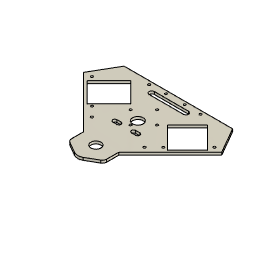
侧板1-正面 v9 (Autodesk Fusion 360 design; units mm, degrees)
Autodesk Fusion 360 part; units mm, degrees
sketch "草图1" plane through (0, 0, 0) normal (0, 0, 1) x (1, 0, 0)
  line L0 (-54.1241, 76.0619) -> (-2.5053, 24.4431)
  line L1 (93.1135, 76.0619) -> (41.4947, 24.4431)
  line L2 (16.6481, 16.6481) -> (19.4947, 16.6481)
  line L3 (-43.8746, 113.133) -> (82.8641, 113.133)
  line L4 (19.4947, 16.6481) -> (19.4947, 38.6817) construction
  line L5 (-2.5053, 4.4431) -> (23.0093, 4.4431) construction
  line L6 (-54.1241, 76.0619) -> (-61.1951, 83.133)
  line L7 (-61.1951, 83.133) -> (-43.8746, 113.133)
  line L8 (-61.1951, 83.133) -> (-22.8991, 83.133) construction
  line L9 (100.1846, 83.133) -> (82.8641, 113.133)
  line L10 (93.1135, 76.0619) -> (100.1846, 83.133)
  line L11 (-2.5053, 24.4431) -> (-1.091, 23.0289)
  line L12 (-1.091, 23.0289) -> (-1.091, 6.0289)
  line L13 (-1.091, 6.0289) -> (19.4947, -5.8563)
  line L14 (19.4947, -5.8563) -> (19.4947, 1) construction
  line L15 (40.0805, 6.0289) -> (19.4947, -5.8563)
  line L16 (40.0805, 23.0289) -> (40.0805, 6.0289)
  line L17 (41.4947, 24.4431) -> (40.0805, 23.0289)
  dimension "d8" = 20
  dimension "d9" = 73
  dimension "d75" = 10
  dimension "d76" = 60
  dimension "d81" = 2
  dimension "d82" = 17
  dimension "d96" = 30
  constraint perpendicular L0 L1
  constraint horizontal L2
  constraint perpendicular L2 L4
  constraint symmetric L0.end L4 L1.end
  constraint horizontal L5
  constraint equal L0 L1
  constraint parallel L0 L6
  constraint horizontal L8
  constraint symmetric L0.start L4 L1.start
  constraint symmetric L4 L6.end L9.start
  constraint symmetric L4 L3.start L3.end
  constraint parallel L0 L11
  constraint perpendicular L5 L12
  constraint vertical L14
  constraint symmetric L0.end L14 L1.end
  constraint symmetric L11.end L14 L16.start
  constraint symmetric L12.end L14 L15.start
  constraint symmetric L13.end L14 L15.end
  measures "d8" distance of L0.end L5.start
  measures "d9" distance of L0.start L0.end
  measures "d75" distance of L0.start L6.end
  measures "d76" angle of L7 L8
  measures "d81" distance of L0.end L11.end
  measures "d82" distance of L11.end L12.end
  measures "d96" distance of L3 L8
extrude "拉伸1" add sketch "草图1" along normal blind 3
sketch "草图2" plane through (0, 0, 3) normal (0, 0, 1) x (-1, 0, 0)
  line L0 (61.1951, -83.133) -> (1.091, -23.0289)
  line L1 (-40.0805, -23.0289) -> (-100.1846, -83.133)
  line L2 (-82.8641, -113.133) -> (43.8746, -113.133)
  line L3 (61.1951, -83.133) -> (56.2454, -88.0827) construction
  line L4 (56.2454, -88.0827) -> (52.0027, -83.8401) construction
  circle A0 centre (52.0027, -83.8401) radius 1.3
  line L5 (52.0027, -83.8401) -> (22.1494, -53.9867) construction
  circle A1 centre (22.1494, -53.9867) radius 1.3
  line L6 (-19.4947, 8.2586) -> (-19.4947, -40) construction
  circle A2 centre (-61.1389, -53.9867) radius 1.3
  circle A3 centre (-90.9922, -83.8401) radius 1.3
  line L7 (-19.4947, -113.133) -> (-19.4947, -109.133) construction
  line L8 (-19.4947, -109.133) -> (-19.4947, -87.1743)
  line L9 (-19.4947, -87.1743) -> (-19.4947, -80.1743) construction
  circle A4 centre (-19.4947, -16.9209) radius 5.95
  line L10 (-90.9922, -83.8401) -> (-75.2591, -68.107) construction
  line L11 (-75.2591, -68.107) -> (-78.0875, -65.2785) construction
  line L12 (-78.0875, -65.2785) -> (-89.7548, -76.9458)
  line L13 (-89.7548, -76.9458) -> (-64.2989, -102.4016)
  line L14 (-64.2989, -102.4016) -> (-53.987, -92.0897)
  line L15 (-40.9644, -79.0671) -> (-51.2764, -89.3791)
  line L16 (-66.4203, -53.6113) -> (-40.9644, -79.0671)
  line L17 (-78.0875, -65.2785) -> (-66.4203, -53.6113)
  line L18 (25.3094, -102.4016) -> (14.9975, -92.0897)
  line L19 (50.7653, -76.9458) -> (25.3094, -102.4016)
  line L20 (39.098, -65.2785) -> (50.7653, -76.9458)
  line L21 (39.098, -65.2785) -> (27.4308, -53.6113)
  line L22 (27.4308, -53.6113) -> (1.9749, -79.0671)
  line L23 (1.9749, -79.0671) -> (12.2869, -89.3791)
  line L24 (-19.4947, -113.133) -> (-19.4947, -109.133)
  line L25 (-19.4947, -109.133) -> (-49.4947, -109.133) construction
  circle A5 centre (-49.4947, -109.133) radius 1.3
  circle A6 centre (10.5053, -109.133) radius 1.3
  line L26 (-19.4947, -113.133) -> (-19.4947, -92.133)
  line L27 (-19.4947, -92.133) -> (3.0053, -92.133) construction
  line L28 (-19.4947, -83.5619) -> (-19.4947, 8.2586) construction
  line L29 (12.2869, -89.3791) -> (-2.5623, -74.5298) construction
  line L30 (14.9975, -92.0897) -> (12.2869, -89.3791)
  line L31 (-53.987, -92.0897) -> (-51.2764, -89.3791)
  line L32 (-19.4947, -72.9209) -> (-10.9947, -72.9209) construction
  circle A7 centre (-19.4947, -65.9209) radius 6.25
  line L33 (-100.1846, -83.133) -> (-82.8641, -113.133)
  line L34 (43.8746, -113.133) -> (61.1951, -83.133)
  line L35 (0.5053, -99.133) -> (-39.4947, -99.133)
  arc A8 (-39.4947, -99.133) -> (-39.4947, -105.133) centre (-39.4947, -102.133) ccw
  line L36 (-39.4947, -105.133) -> (0.5053, -105.133)
  arc A9 (0.5053, -105.133) -> (0.5053, -99.133) centre (0.5053, -102.133) ccw
  line L37 (0.5053, -102.133) -> (-39.4947, -102.133) construction
  line L38 (43.8746, -113.133) -> (-82.8641, -113.133)
  line L39 (1.091, -23.0289) -> (1.091, -6.0289)
  line L40 (1.091, -6.0289) -> (-19.4947, 5.8563)
  line L41 (-19.4947, 5.8563) -> (-40.0805, -6.0289)
  line L42 (-40.0805, -6.0289) -> (-40.0805, -23.0289)
  line L43 (-19.4947, -65.9209) -> (-19.4947, -72.9209)
  circle A10 centre (-19.4947, -72.9209) radius 15.5 construction
  circle A11 centre (-19.4947, -57.4209) radius 1.3
  circle A12 centre (-19.4947, -88.4209) radius 1.3
  circle A13 centre (-19.4947, -72.9209) radius 18.5 construction
  circle A14 centre (-3.9947, -72.9209) radius 1.3
  circle A15 centre (-34.9947, -72.9209) radius 1.3
  line L44 (22.1494, -53.9867) -> (11.1892, -43.0266)
  circle A16 centre (11.1892, -43.0266) radius 1.4
  circle A17 centre (-50.1787, -43.0266) radius 1.4
  line L45 (-19.4947, -65.9209) -> (-32.9298, -52.4858) construction
  line L46 (-19.4947, -65.9209) -> (-1.4947, -65.9209) construction
  line L47 (-32.9298, -54.8858) -> (-27.9298, -54.8858)
  arc A18 (-27.9298, -54.8858) -> (-27.9298, -50.0858) centre (-27.9298, -52.4858) ccw
  line L48 (-27.9298, -50.0858) -> (-32.9298, -50.0858)
  arc A19 (-32.9298, -50.0858) -> (-32.9298, -54.8858) centre (-32.9298, -52.4858) ccw
  line L49 (-32.9298, -52.4858) -> (-27.9298, -52.4858) construction
  arc A20 (-32.9298, -50.0858) -> (-32.9298, -54.8858) centre (-32.9298, -52.4858) ccw
  arc A21 (-11.0597, -50.0858) -> (-11.0597, -54.8858) centre (-11.0597, -52.4858) ccw
  line L50 (-6.0597, -54.8858) -> (-11.0597, -54.8858)
  arc A22 (-6.0597, -54.8858) -> (-6.0597, -50.0858) centre (-6.0597, -52.4858) ccw
  line L51 (-11.0597, -50.0858) -> (-6.0597, -50.0858)
  line L52 (-19.4947, -109.133) -> (-8.4947, -109.133) construction
  line L53 (-8.4947, -113.133) -> (-8.4947, -109.633) construction
  circle A23 centre (-8.4947, -109.633) radius 1.3
  circle A24 centre (-30.4947, -109.633) radius 1.3
  point P0 (-19.4947, -102.133)
  dimension "d10" = 7
  dimension "d11" = 6
  dimension "d12" = 2.6
  dimension "d13" = 42.219
  dimension "d14" = 2.6
  dimension "d19" = 7
  dimension "d23" = 11.9
  dimension "d26" = 22.25
  dimension "d28" = 4
  dimension "d29" = 16.5
  dimension "d30" = 36
  dimension "d40" = 30
  dimension "d41" = 2.6
  dimension "d45" = 21
  dimension "d46" = 22.5
  dimension "d63" = 21
  dimension "d70" = 12.5
  dimension "d77" = 6
  dimension "d78" = 8
  dimension "d87" = 49
  dimension "d88" = 7
  dimension "d89" = 31
  dimension "d90" = 2.6
  dimension "d92" = 360
  dimension "d93" = 37
  dimension "d97" = 2.6
  dimension "d98" = 2.6
  dimension "d101" = 15.5
  dimension "d102" = 2.8
  dimension "d105" = 135
  dimension "d106" = 19
  dimension "d107" = 4.8
  dimension "d110" = 5
  dimension "d113" = 11
  dimension "d117" = 4
  dimension "d118" = 3.5
  dimension "d119" = 2.6
  constraint coincident L0.start L3.start
  constraint perpendicular L0 L3
  constraint perpendicular L3 L4
  constraint coincident L4.end A0.centre
  constraint parallel L4 L5
  constraint coincident L5.end A1.centre
  constraint vertical L6
  constraint symmetric A0 L6 A3
  constraint symmetric A1 L6 A2
  constraint midpoint L2 L7.start
  constraint perpendicular L2 L7
  constraint parallel L7 L8
  constraint vertical L9
  constraint coincident L6 A4.centre
  constraint coincident A3.centre L10.start
  constraint perpendicular L10 L11
  constraint perpendicular L11 L12
  constraint perpendicular L10 L13
  constraint perpendicular L13 L14
  constraint symmetric L12.start L11 L17.start
  constraint symmetric L11 L12.end L16.start
  constraint symmetric L11 L13.end L15.start
  constraint symmetric L11 L14.end L15.end
  constraint symmetric L6 L11.end L20.start
  constraint symmetric L6 L12.end L19.start
  constraint symmetric L6 L13.end L18.start
  constraint symmetric L6 L14.end L18.end
  constraint symmetric L6 L15.start L22.end
  constraint symmetric L6 L15.end L23.end
  constraint symmetric L6 L16.start L21.end
  constraint perpendicular L2 L24
  constraint perpendicular L8 L25
  constraint coincident L25.end A5.centre
  constraint symmetric L7 A5 A6
  constraint perpendicular L2 L26
  constraint perpendicular L26 L27
  constraint perpendicular L22 L29
  constraint parallel L29 L30
  constraint perpendicular L23 L31
  constraint perpendicular L28 L32
  constraint tangent L35 A8
  constraint tangent A8 L36
  constraint parallel L35 L36
  constraint tangent L36 A9
  constraint tangent L35 A9
  constraint perpendicular L8 L37
  constraint coincident L8 P0
  constraint midpoint L37 P0
  constraint coincident A7.centre L43.start
  constraint perpendicular L27 L43
  constraint coincident L32.start L43.end
  constraint coincident A10 A11.centre
  constraint coincident L28 A11.centre
  constraint coincident A10 A14.centre
  constraint coincident A10 A15.centre
  constraint perpendicular L22 L44
  constraint coincident L44.end A16.centre
  constraint symmetric L28 A16 A17
  constraint horizontal L46
  constraint coincident L45.end A19.centre
  constraint tangent L47 A18
  constraint tangent A18 L48
  constraint parallel L47 L48
  constraint tangent L48 A19
  constraint tangent L47 A19
  constraint horizontal L49
  constraint symmetric L28 L47.start L50.start
  constraint symmetric L28 L47.end A21.end
  constraint symmetric L28 A18.end A21.start
  constraint symmetric L28 L48.end A22.end
  constraint symmetric L28 A18 A21
  constraint symmetric L28 A20 A22
  constraint perpendicular L7 L52
  constraint coincident L38 L53.start
  constraint perpendicular L52 L53
  constraint coincident L53.end A23.centre
  constraint symmetric L8 A23 A24
  measures "d10" distance of L0.start L3.end
  measures "d11" distance of L3.end L4.end
  measures "d12" diameter of A0
  measures "d13" distance of L4.end L5.end
  measures "d14" diameter of A1
  measures "d19" distance of L8.end L9.end
  measures "d23" diameter of A4
  measures "d26" distance of A3.centre L10.end
  measures "d28" distance of L10.end L11.end
  measures "d29" distance of L11.end L12.end
  measures "d30" distance of L12.end L13.end
  measures "d40" distance of L7.end L25.end
  measures "d41" diameter of A5
  measures "d45" distance of L7.start L26.end
  measures "d46" distance of L26.end L27.end
  measures "d63" distance of L23.end L29.end
  measures "d70" diameter of A7
  measures "d77" diameter of A8
  measures "d78" distance of L36 L38
  measures "d87" distance of A4.centre A7.centre
  measures "d88" distance of A7.centre L32.start
  measures "d89" diameter of A10
  measures "d90" diameter of A11
  measures "d93" diameter of A13
  measures "d97" diameter of A14
  measures "d98" diameter of A15
  measures "d101" distance of L5.end L44.end
  measures "d102" diameter of A16
  measures "d105" angle of L45 L46
  measures "d106" distance of A7.centre L45.end
  measures "d107" diameter of A20
  measures "d110" distance of L45.end A18.centre
  measures "d113" distance of L7.end L52.end
  measures "d117" distance of A6.centre L38
  measures "d118" distance of L53.start L53.end
  measures "d119" diameter of A23
extrude "拉伸2" cut sketch "草图2" against normal blind 3 contours A0 | A1 | A2 | A3
extrude "拉伸4" cut sketch "草图2" against normal blind 3 contours A4
extrude "拉伸6" cut sketch "草图2" against normal blind 3 contours A5 | A6
extrude "拉伸9" cut sketch "草图2" against normal blind 3 contours L12 L13 L14 L15 L16 L17 L31 | L18 L19 L20 L21 L22 L23 L30
extrude "拉伸10" cut sketch "草图2" against normal blind 3 contours A7
extrude "拉伸11" cut sketch "草图2" against normal blind 3 contours L8 L26 L35 A8 L36 | L8 L26 L35 L36 A9
fillet "圆角4" radius 10 1 edges at (19.4947, -5.8563, 1.5)
fillet "圆角5" radius 5 2 edges at (40.0805, 6.0289, 1.5) (-1.091, 6.0289, 1.5)
extrude "拉伸12" cut sketch "草图2" against normal blind 3 contours A11 | A12
extrude "拉伸13" cut sketch "草图2" against normal blind 3 contours A14 | A15
extrude "拉伸14" cut sketch "草图2" against normal blind 3 contours A16 | A17
extrude "拉伸15" cut sketch "草图2" against normal blind 3 contours L47 A18 L48 A19 A20
extrude "拉伸16" cut sketch "草图2" against normal blind 3 contours A21 L50 A22 L51
extrude "拉伸18" cut sketch "草图2" against normal blind 3 contours A23 | A24
equation "d46 = ( 45 / 2 ) * 1 mm"
equation "d63 = ( 42 / 2 ) * 1 mm"
equation "d87 = 48.5 mm + 0.5 mm"
equation "d113 = ( 22 / 2 ) * 1 mm"
